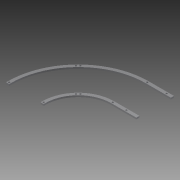
# Autodesk Inventor part: Runner Rails v1
Saved by Autodesk Inventor 2013 (Build 170138000, 138)
## iProperties
Created: 2013-01-15
Part Number: Runner Rails v1
Material: Polycarbonate, Clear
Document SubType Name: Modeling
Designer: actoennies
Mass: 60.9931 g
Surface Area: 342.612 cm^2
Volume: 68.2249 cm^3
Density: 0.894 g/cm^3
Author: actoennies
Autodesk Inventor part; units mm, degrees
ref_plane "YZ Plane" through (0, 0, 0) normal (1, 0, 0) x (0, 1, 0)
ref_plane "XZ Plane" through (0, 0, 0) normal (0, 1, 0) x (-1, 0, 0)
ref_plane "XY Plane" through (0, 0, 0) normal (0, 0, 1) x (1, 0, 0)
sketch "Sketch1" plane through (0, 0, 0) normal (0, 1, 0) x (-1, 0, 0)
  arc A0 (0, -273.05) -> (273.05, 0) centre (0, 0) ccw
  arc A1 (0, -285.75) -> (285.75, 0) centre (0, 0) ccw
  line L0 (-101.6, -133.35) -> (0, -133.35)
  line L1 (-101.6, -146.05) -> (-101.6, -133.35)
  line L2 (0, -146.05) -> (-101.6, -146.05)
  arc A2 (0, -146.05) -> (146.05, 0) centre (0, 0) ccw
  arc A3 (0, -133.35) -> (133.35, 0) centre (0, 0) ccw
  line L3 (-101.6, -273.05) -> (0, -273.05)
  line L4 (0, -285.75) -> (-101.6, -285.75)
  line L5 (146.05, 0) -> (146.05, 6.35)
  line L6 (133.35, 0) -> (133.35, 6.35)
  line L7 (273.05, 6.35) -> (273.05, 0)
  line L8 (285.75, 6.35) -> (285.75, 0)
  line L9 (-101.6, -285.75) -> (-101.6, -273.05)
  circle A4 centre (103.1708, -94.1906) radius 3.3782
  circle A5 centre (94.1906, -103.1708) radius 3.3782
  circle A6 centre (279.4, 0) radius 3.3782
  circle A7 centre (139.7, 0) radius 3.3782
  circle A8 centre (202.0047, -193.0245) radius 3.3782
  circle A9 centre (193.0245, -202.0047) radius 3.3782
  circle A10 centre (0, -279.4) radius 3.3782
  circle A11 centre (0, -139.7) radius 3.3782
  circle A12 centre (-55.2746, -139.7) radius 3.3782
  circle A13 centre (-78.3684, -279.4) radius 3.3782
  line L10 (285.75, 6.35) -> (273.05, 6.35)
  line L11 (146.05, 6.35) -> (133.35, 6.35)
  dimension "d10" = 12.7
  dimension "d11" = 12.7
  dimension "d13" = 12.7
  dimension "d14" = 6.7564
  dimension "d15" = 6.7564
  dimension "d16" = 6.7564
  dimension "d18" = 6.7564
  dimension "d20" = 6.35
  dimension "d21" = 6.7564
  dimension "d22" = 6.7564
  dimension "d23" = 6.7564
  dimension "d24" = 6.35
  dimension "d26" = 6.7564
  dimension "d27" = 6.35
  dimension "d30" = 6.7564
  dimension "d31" = 6.35
  dimension "d32" = 6.7564
  dimension "d33" = 6.35
  constraints: 24 end point, 14 centre point, 8 point on circle, 4 tangent, 3 coincident, 3 equal length, 3 perpendicular
  measures "d10" distance between parallel lines of L5 L6
  measures "d11" distance between parallel lines of L7 L8
  measures "d13" distance of L1.start L0.start
  measures "d14" diameter of A4
  measures "d15" diameter of A5
  measures "d16" diameter of A6
  measures "d18" diameter of A7
  measures "d20" distance from line of L5 A7.centre
  measures "d21" diameter of A8
  measures "d22" diameter of A9
  measures "d23" diameter of A10
  measures "d24" distance from line of L3 A10.centre
  measures "d26" diameter of A11
  measures "d27" distance from line of L0 A11.centre
  measures "d30" diameter of A12
  measures "d31" distance from line of L0 A12.centre
  measures "d32" diameter of A13
  measures "d33" distance from line of L3 A13.centre
extrude "Extrusion1" add sketch "Sketch1" along normal blind 6.35
body "Solid1"
